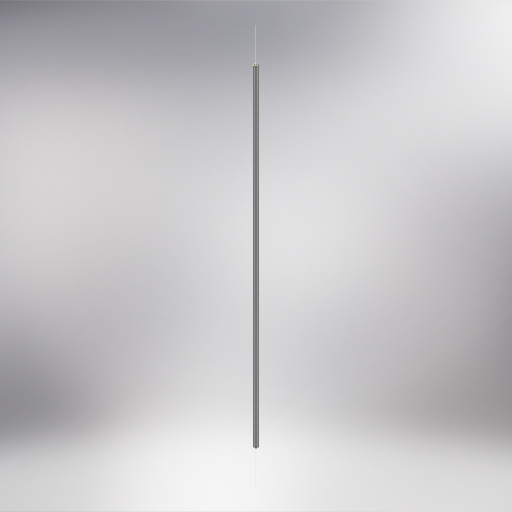
# Autodesk Inventor part: 12inch shaft
Saved by Autodesk Inventor 2023 (Build 270158000, 158)
## iProperties
Created: 2023-03-24
Part Number: 12inch shaft
Material: Stainless Steel
Document SubType Name: Modeling
Designer: aaron
Density: 8 g/cm^3
Appearance: Semi-Polished
Author: aaron
Autodesk Inventor part; units mm, degrees
ref_plane "YZ Plane" through (0, 0, 0) normal (1, 0, 0) x (0, 1, 0)
ref_plane "XZ Plane" through (0, 0, 0) normal (0, 1, 0) x (-1, 0, 0)
ref_plane "XY Plane" through (0, 0, 0) normal (0, 0, 1) x (1, 0, 0)
sketch "Sketch1" plane through (0, 0, 0) normal (0, 1, 0) x (-1, 0, 0)
  line L0 (-1.5875, -1.5875) -> (1.5875, -1.5875)
  line L1 (1.5875, -1.5875) -> (1.5875, 1.5875)
  line L2 (1.5875, 1.5875) -> (-1.5875, 1.5875)
  line L3 (-1.5875, 1.5875) -> (-1.5875, -1.5875)
  line L4 (-1.5875, -1.5875) -> (1.5875, 1.5875) construction
  line L5 (1.5875, -1.5875) -> (-1.5875, 1.5875) construction
  point P0 (0, 0)
  dimension "d0" = 3.175
  dimension "d1" = 3.175
  constraints: 12 end point, 2 midpoint, 2 parallel, 1 horizontal, 1 perpendicular
  measures "d0" distance of L2.end L1.end
  measures "d1" distance of L1.end L0.end
extrude "Extrusion1" add sketch "Sketch1" along normal blind 304.8
fillet "Fillet1" radius 0.7937 4 edges at (1.5875, 152.4, -1.5875) (-1.5875, 152.4, -1.5875) (1.5875, 152.4, 1.5875) (-1.5875, 152.4, 1.5875)
fillet "Fillet2" radius 0.3969 16 edges at (1.5875, 0, 0) (1.355, 0, -1.355) (0, 0, -1.5875) (-1.355, 0, -1.355) (-1.5875, 0, 0) (-1.355, 0, 1.355) (0, 0, 1.5875) (1.355, 0, 1.355) (0, 304.8, 1.5875) (-1.355, 304.8, 1.355) (-1.5875, 304.8, 0) (-1.355, 304.8, -1.355) (0, 304.8, -1.5875) (1.355, 304.8, -1.355) (1.5875, 304.8, 0) (1.355, 304.8, 1.355)
body "Solid1"
